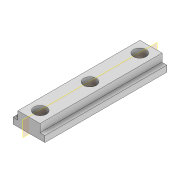
# Autodesk Inventor part: 585757_plastic_1061_holes
Saved by Autodesk Inventor 2020 (Build 240168000, 168)
## iProperties
Created: 2020-01-02
Part Number: 585757_plastic_1061_holes
Material: Generic
Document SubType Name: Modeling
Designer: ball
Density: 1 g/cm^3
Appearance: Default
Author: ball
Autodesk Inventor part; units mm, degrees
ref_plane "XZ Plane" through (0, 0, 0) normal (0, 1, 0) x (-1, 0, 0)
ref_plane "XY Plane" through (0, 0, 0) normal (0, 0, 1) x (1, 0, 0)
sketch "Sketch1" plane through (0, 0, 0) normal (0, 1, 0) x (-1, 0, 0)
  line L0 (4.318, 16.51) -> (-4.318, 16.51)
  line L1 (-4.318, 16.51) -> (-4.318, -16.51)
  line L2 (-4.318, -16.51) -> (4.318, -16.51)
  line L3 (4.318, -16.51) -> (4.318, 16.51)
  line L4 (4.318, 16.51) -> (-4.318, -16.51) construction
  line L5 (-4.318, 16.51) -> (4.318, -16.51) construction
  point P0 (0, 0)
  dimension "d0" = 8.636
  dimension "d1" = 33.02
  constraints: 12 end point, 2 midpoint, 2 parallel, 1 horizontal, 1 perpendicular
  measures "d0" distance of L2.end L1.end
  measures "d1" distance of L1.end L0.end
extrude "Base" add sketch "Sketch1" along normal blind 1.651
sketch "Sketch2" plane through (0, 1.651, 0) normal (0, 1, 0) x (1, 0, 0)
  line L0 (-2.9972, -16.51) -> (2.9972, -16.51)
  line L1 (2.9972, -16.51) -> (2.9972, 16.51)
  line L2 (2.9972, 16.51) -> (-2.9972, 16.51)
  line L3 (-2.9972, 16.51) -> (-2.9972, -16.51)
  line L4 (-2.9972, -16.51) -> (2.9972, 16.51) construction
  line L5 (2.9972, -16.51) -> (-2.9972, 16.51) construction
  point P0 (0, 0)
  dimension "d4" = 5.9944
  dimension "d5" = 33.02
  constraints: 12 end point, 2 midpoint, 2 parallel, 1 horizontal, 1 perpendicular
  measures "d4" distance of L2.end L1.end
  measures "d5" distance of L1.end L0.end
extrude "Step" add sketch "Sketch2" along normal blind 2.159
sketch "Sketch3" plane through (0, 3.81, 0) normal (0, 1, 0) x (1, 0, 0)
  circle A0 centre (0, 0) radius 1.7018
  circle A1 centre (0, -13.4747) radius 1.7018
  circle A2 centre (0, 13.4747) radius 1.7018
  dimension "d8" = 3.4036
  dimension "d9" = 3.4036
  dimension "d10" = 3.4036
  dimension "d11" = 13.4747
  dimension "d12" = 13.4747
  constraints: 3 centre point, 1 coincident
  measures "d8" diameter of A0
  measures "d9" diameter of A1
  measures "d10" diameter of A2
  measures "d11" distance of A1.centre point (0, 0)
  measures "d12" distance of A2.centre point (0, 0)
extrude "Holes" cut sketch "Sketch3" against normal through all
equation "\"d11\" = d12"
body "Solid1"
